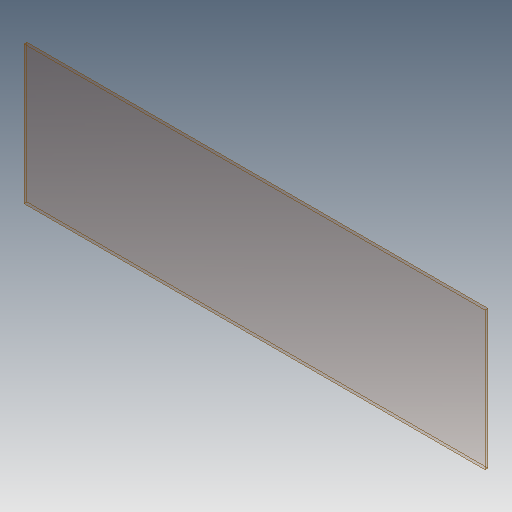
# Autodesk Inventor part: wallPlate
Saved by Autodesk Inventor 2018 (Build 220112000, 112)
## iProperties
Created: 2017-04-19
Part Number: wallPlate
Material: Polycarbonate, Smoke
Document SubType Name: Modeling
Designer: sawaiz
Density: 1.2 g/cm^3
Appearance: Polycarbonate - Smoked
Author: sawaiz
Autodesk Inventor part; units mm, degrees
ref_plane "YZ Plane" through (0, 0, 0) normal (1, 0, 0) x (0, 1, 0)
ref_plane "XZ Plane" through (0, 0, 0) normal (0, 1, 0) x (-1, 0, 0)
ref_plane "XY Plane" through (0, 0, 0) normal (0, 0, 1) x (1, 0, 0)
sketch "Sketch2" plane through (0, 0, 0) normal (0, 0, 1) x (1, 0, 0)
  line L0 (-250, -75) -> (250, -75)
  line L1 (250, -75) -> (250, 75)
  line L2 (250, 75) -> (-250, 75)
  line L3 (-250, 75) -> (-250, -75)
  line L4 (-250, -75) -> (250, 75) construction
  line L5 (250, -75) -> (-250, 75) construction
  point P0 (0, 0)
  dimension "d1" = 500
  dimension "d2" = 150
  constraints: 12 end point, 2 midpoint, 2 parallel, 1 horizontal, 1 perpendicular
  measures "d1" distance of L2.end L1.end
  measures "d2" distance of L1.end L0.end
extrude "Extrusion1" add sketch "Sketch2" along normal mid plane 3.125
equation "\"d1\" = 0.5 * depth"
equation "\"d2\" = height"
equation "\"d3\" = acrylicThickness"
equation "\"height\" = 150"
equation "\"acrylicThickness\" = 3.125"
equation "\"depth\" = 1000"
body "Solid1"
